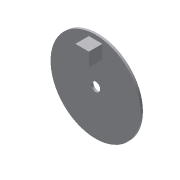
# Autodesk Inventor part: Black shipping good
Saved by Autodesk Inventor 2015 (Build 190159000, 159)
## iProperties
Created: 2015-03-07
Part Number: Black shipping good
Material: Generic
Document SubType Name: Modeling
Designer: Vukica
Density: 1 g/cm^3
Appearance: Default
Author: Vukica
Autodesk Inventor part; units mm, degrees
ref_plane "YZ Plane" through (0, 0, 0) normal (1, 0, 0) x (0, 1, 0)
ref_plane "XZ Plane" through (0, 0, 0) normal (0, 1, 0) x (-1, 0, 0)
ref_plane "XY Plane" through (0, 0, 0) normal (0, 0, 1) x (1, 0, 0)
sketch "Sketch1" plane through (0, 0, 0) normal (0, 0, 1) x (1, 0, 0)
  circle A0 centre (0, 0) radius 63.5
  circle A1 centre (0, 0) radius 6.35
  dimension "d0" = 127
  dimension "d1" = 12.7
  constraints: 2 centre point, 2 coincident
  measures "d0" diameter of A0
  measures "d1" diameter of A1
extrude "Extrusion1" add sketch "Sketch1" along normal blind 3.175
sketch "Sketch2" plane through (0, 0, 3.175) normal (0, 0, 1) x (1, 0, 0)
  circle A0 centre (0, 0) radius 6.35 construction
  line L0 (0, 0) -> (0, 98.5541) construction
  line L1 (-9.525, 57.15) -> (9.525, 57.15)
  line L2 (9.525, 57.15) -> (9.525, 38.1)
  line L3 (9.525, 38.1) -> (-9.525, 38.1)
  line L4 (-9.525, 38.1) -> (-9.525, 57.15)
  line L5 (0, 0) -> (107.2184, 0) construction
  dimension "d4" = 38.1
  dimension "d5" = 19.05
  dimension "d6" = 19.05
  constraints: 12 end point, 3 horizontal, 2 parallel, 2 vertical, 1 perpendicular, 1 other
  measures "d4" distance between parallel lines of L5 L3
  measures "d5" distance of L1.start L1.end
  measures "d6" distance of L3.end L1.start
extrude "Extrusion2" add sketch "Sketch2" along normal blind 19.05
body "Solid1"
